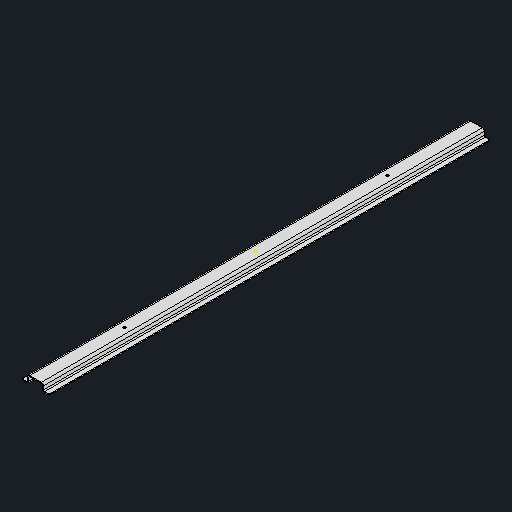
# Autodesk Inventor part: 5th Wheel Hitch Sliding rail
Saved by Autodesk Inventor 2025.1 (Build 291241000, 241)
## iProperties
Created: 2026-02-24
Part Number: 5th Wheel Hitch Sliding rail
Material: Generic
Document SubType Name: Sheet Metal
Designer: Desktop -24
Density: 1 g/cm^3
Flat Pattern Width: 17.0103 cm
Flat Pattern Length: 203.2 cm
Flat Pattern Area: 3456.5 cm^2
Sheet Metal Rule: Default
Sheet Metal Width: 6.697 in
Sheet Metal Length: 80.000 in
Sheet Metal Area: 535.759 in^2
Appearance: Default
Author: Desktop -24
Autodesk Inventor part; units mm, degrees
ref_plane "YZ Plane" through (0, 0, 0) normal (1, 0, 0) x (0, 1, 0)
ref_plane "XZ Plane" through (0, 0, 0) normal (0, 1, 0) x (-1, 0, 0)
ref_plane "XY Plane" through (0, 0, 0) normal (0, 0, 1) x (1, 0, 0)
sketch "Sketch1" plane through (0, 0, 0) normal (0, 0, 1) x (1, 0, 0)
  point P0 (0, 0)
sketch "Sketch2" plane through (0, 0, 0) normal (0, 1, 0) x (-1, 0, 0)
  line L0 (-31.75, 1016) -> (31.75, 1016)
  line L1 (31.75, 1016) -> (31.75, -1016)
  line L2 (31.75, -1016) -> (-31.75, -1016)
  line L3 (-31.75, -1016) -> (-31.75, 1016)
  line L4 (-31.75, 1016) -> (31.75, -1016) construction
  line L5 (31.75, 1016) -> (-31.75, -1016) construction
  line L6 (0, -1016) -> (0, 1016)
  point P0 (0, 0)
  point P1 (0, -657.225)
  point P2 (0, -606.425)
  point P3 (0, 657.225)
  point P4 (0, 606.425)
  point P5 (0, 0)
  dimension "d0" = 63.5
  dimension "d1" = 2032
  dimension "d24" = 50.8
  dimension "d26" = 50.8
  dimension "d27" = 1212.85
  dimension "d28" = 606.425
  constraints: 14 end point, 5 midpoint, 4 point on line, 2 parallel, 1 horizontal, 1 perpendicular
  measures "d0" distance of L1.end L2.end
  measures "d1" distance of L2.end L0.start
  measures "d24" distance of point (0, 606.425) point (0, 657.225)
  measures "d26" distance of point (0, -657.225) point (0, -606.425)
  measures "d27" distance of point (0, 606.425) point (0, -606.425)
  measures "d28" distance of point (0, 0) point (0, 606.425)
extrude "Plate1" add sketch "Sketch2" against normal blind 4.7752
sketch "Sketch3" plane through (36.5252, 0, 1016) normal (-1, 0, 0) x (0, -1, 0)
  line L0 (0, -2032) -> (0, 0)
  line L1 (0, 0) -> (30.1752, 0)
  line L2 (30.1752, 0) -> (30.1752, -2032)
  line L3 (30.1752, -2032) -> (0, -2032)
  constraints: 8 end point
edge flange "Flange1" height 25.4 angle 90 thickness 4.7752 bend radius 4.7752 thickness toward (-1, 0, 0) relief tear relief width 4.7752 relief depth 2.3876 corner gap 4.7752 corner form 0 edges at (31.75, -4.7752, 0) (-31.75, -4.7752, 0) wall of the first edge with corners at (36.5252, 0, -1016) (36.5252, 0, 1016) (36.5252, -30.1752, 1016) (36.5252, -30.1752, -1016)
bend "Bend1"
corner "Corner1"
sketch "Sketch4" plane through (31.75, -34.9504, -1016) normal (0, 1, 0) x (-1, 0, 0)
  line L0 (0, 2032) -> (0, 0)
  line L1 (0, 0) -> (-30.1752, 0)
  line L2 (-30.1752, 0) -> (-30.1752, 2032)
  line L3 (-30.1752, 2032) -> (0, 2032)
  constraints: 8 end point
edge flange "Flange2" height 25.4 angle 90 thickness 4.7752 bend radius 4.7752 thickness toward (0, 1, 0) relief tear relief width 4.7752 relief depth 2.3876 corner gap 4.7752 corner form 0 edges at (36.5252, -30.1752, 0) (-36.5252, -30.1752, 0) wall of the first edge with corners at (31.75, -34.9504, 1016) (31.75, -34.9504, -1016) (61.9252, -34.9504, -1016) (61.9252, -34.9504, 1016)
bend "Bend2"
corner "Corner2"
hole "Hole1" at (0, 0, 606.425) at (0, 0, -606.425) direction (0, -1, 0) diameter 12.7 end through all
fillet "Corner Round1" radius 6.35 4 edges at (61.9252, -32.5628, 1016) (-61.9252, -32.5628, 1016) (-61.9252, -32.5628, -1016) (61.9252, -32.5628, -1016)
equation "\"d28\" = 0.5 * d27"
equation "\"d34\" = Thickness"
equation "\"d2\" = Thickness"
equation "\"d3\" = BendReliefWidth"
equation "\"d4\" = BendReliefDepth"
equation "\"d5\" = MinimumRemnant"
equation "\"d6\" = TransitionRadius"
equation "\"d9\" = BendRadius"
equation "\"d10\" = CornerReliefSize"
equation "\"d11\" = GapSize"
equation "\"d12\" = JacobiRadiusSize"
equation "\"d13\" = BendReliefWidth"
equation "\"d14\" = BendReliefDepth"
equation "\"d15\" = MinimumRemnant"
equation "\"d16\" = TransitionRadius"
equation "\"d19\" = BendRadius"
equation "\"d20\" = CornerReliefSize"
equation "\"d21\" = GapSize"
equation "\"d22\" = JacobiRadiusSize"
equation "\"BendRadius\" = Thickness"
equation "\"BendReliefWidth\" = Thickness"
equation "\"BendReliefDepth\" = 0.5 * Thickness"
equation "\"CornerReliefSize\" = 4 * Thickness"
equation "\"MinimumRemnant\" = 2 * Thickness"
equation "\"TransitionRadius\" = BendRadius"
equation "\"JacobiRadiusSize\" = BendRadius"
equation "\"GapSize\" = Thickness"
equation "\"Thickness\" = 4.7752"
body "Solid1"
